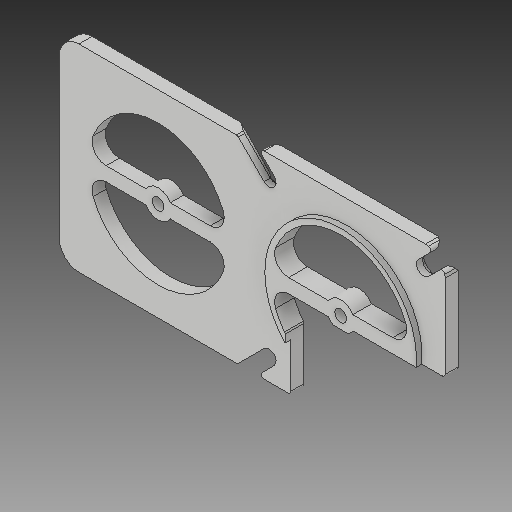
# Autodesk Inventor part: V4 in walldual
Saved by Autodesk Inventor 2020 (Build 240168000, 168)
## iProperties
Created: 2020-01-08
Part Number: V4 in walldual
Material: Generic
Document SubType Name: Modeling
Designer: user
Density: 1 g/cm^3
Appearance: Default
Author: user
Autodesk Inventor part; units mm, degrees
ref_plane "YZ Plane" through (0, 0, 0) normal (1, 0, 0) x (0, 1, 0)
ref_plane "XZ Plane" through (0, 0, 0) normal (0, 1, 0) x (-1, 0, 0)
ref_plane "XY Plane" through (0, 0, 0) normal (0, 0, 1) x (1, 0, 0)
sketch "Sketch1" plane through (0, 0, 0) normal (0, 0, 1) x (1, 0, 0)
  line L0 (-95.2, -35.2) -> (28.2, -35.2)
  line L1 (35.2, -28.2) -> (35.2, 28.2)
  line L2 (28.2, 35.2) -> (-95.2, 35.2)
  line L3 (-102.2, 28.2) -> (-102.2, -28.2)
  arc A0 (-95.2, 35.2) -> (-102.2, 28.2) centre (-95.2, 28.2) ccw
  arc A1 (35.2, 28.2) -> (28.2, 35.2) centre (28.2, 28.2) ccw
  arc A2 (-102.2, -28.2) -> (-95.2, -35.2) centre (-95.2, -28.2) ccw
  arc A3 (28.2, -35.2) -> (35.2, -28.2) centre (28.2, -28.2) ccw
  line L4 (24.8747, -2.5) -> (24.8747, 2.5) construction
  line L5 (-24.8747, 2.5) -> (-24.8747, -2.5) construction
  line L6 (24.8747, -2.5) -> (-24.8747, 2.5) construction
  line L7 (24.8747, 2.5) -> (-24.8747, -2.5) construction
  arc A4 (-23.1756, -9.375) -> (23.1756, -9.375) centre (0, 0) ccw
  arc A5 (23.1756, 9.375) -> (-23.1756, 9.375) centre (0, 0) ccw
  arc A6 (-18.5405, -2.5) -> (-23.1756, -9.375) centre (-18.5405, -7.5) ccw
  arc A7 (-23.1756, 9.375) -> (-18.5405, 2.5) centre (-18.5405, 7.5) ccw
  arc A8 (23.1756, -9.375) -> (18.5405, -2.5) centre (18.5405, -7.5) ccw
  arc A9 (18.5405, 2.5) -> (23.1756, 9.375) centre (18.5405, 7.5) ccw
  line L8 (-4.3301, 2.5) -> (-18.5405, 2.5)
  line L9 (-18.5405, -2.5) -> (-4.3301, -2.5)
  line L10 (4.3301, -2.5) -> (18.5405, -2.5)
  line L11 (18.5405, 2.5) -> (4.3301, 2.5)
  arc A10 (-4.3301, -2.5) -> (4.3301, -2.5) centre (0, 0) ccw
  arc A11 (4.3301, 2.5) -> (-4.3301, 2.5) centre (0, 0) ccw
  line L12 (-18.5405, 7.5) -> (18.5405, 7.5) construction
  line L13 (18.5405, -7.5) -> (-18.5405, -7.5) construction
  line L14 (0, 0) -> (0, -35.2) construction
  line L15 (0, 0) -> (0, 35.2) construction
  line L16 (0, 0) -> (35.2, 0) construction
  line L17 (-33.5, -35.2) -> (-33.5, 35.2) construction
  arc A12 (-90.1756, -9.375) -> (-43.8244, -9.375) centre (-67, 0) ccw
  arc A13 (-43.8244, 9.375) -> (-90.1756, 9.375) centre (-67, 0) ccw
  arc A14 (-43.8244, -9.375) -> (-48.4595, -2.5) centre (-48.4595, -7.5) ccw
  arc A15 (-48.4595, 2.5) -> (-43.8244, 9.375) centre (-48.4595, 7.5) ccw
  arc A16 (-85.5405, -2.5) -> (-90.1756, -9.375) centre (-85.5405, -7.5) ccw
  arc A17 (-90.1756, 9.375) -> (-85.5405, 2.5) centre (-85.5405, 7.5) ccw
  line L18 (-62.6699, 2.5) -> (-48.4595, 2.5)
  line L19 (-48.4595, -2.5) -> (-62.6699, -2.5)
  line L20 (-71.3301, -2.5) -> (-85.5405, -2.5)
  line L21 (-85.5405, 2.5) -> (-71.3301, 2.5)
  arc A18 (-71.3301, -2.5) -> (-62.6699, -2.5) centre (-67, 0) ccw
  arc A19 (-62.6699, 2.5) -> (-71.3301, 2.5) centre (-67, 0) ccw
  point P0 (0, 0)
  point P1 (0, 0)
  dimension "d63" = 67
  dimension "d1" = 7
  dimension "d3" = 5
  dimension "d4" = 25
  dimension "d5" = 5
  dimension "d7" = 5
  dimension "d59" = 70.4
  dimension "d60" = 137.4
  constraints: 44 end point, 44 point on circle, 20 centre point, 20 tangent, 18 symmetric about line, 7 equal radius, 7 midpoint, 7 parallel, 5 point on line, 4 horizontal, 3 coincident, 3 perpendicular, 2 equal length, 1 vertical, 9 other
  measures "d1" radius of A0
  measures "d3" distance of L5.end L5.start
  measures "d4" radius of A5
  measures "d5" radius of A6
  measures "d7" radius of A11
  measures "d59" distance between parallel lines of L0 L2
  measures "d60" distance between parallel lines of L3 L1
extrude "Extrusion1" add sketch "Sketch1" along normal blind 4.7
sketch "Sketch2" plane through (0, 0, 4.7) normal (0, 0, 1) x (1, 0, 0)
  circle A0 centre (0, 0) radius 27
  arc A1 (23.1756, 9.375) -> (-23.1756, 9.375) centre (0, 0) ccw projected
  arc A2 (18.5405, 2.5) -> (23.1756, 9.375) centre (18.5405, 7.5) ccw projected
  line L0 (18.5405, 2.5) -> (4.3301, 2.5) projected
  arc A3 (4.3301, 2.5) -> (-4.3301, 2.5) centre (0, 0) ccw projected
  line L1 (-4.3301, 2.5) -> (-18.5405, 2.5) projected
  arc A4 (-23.1756, 9.375) -> (-18.5405, 2.5) centre (-18.5405, 7.5) ccw projected
  line L2 (-18.5405, -2.5) -> (-4.3301, -2.5) projected
  arc A5 (-4.3301, -2.5) -> (4.3301, -2.5) centre (0, 0) ccw projected
  line L3 (4.3301, -2.5) -> (18.5405, -2.5) projected
  arc A6 (23.1756, -9.375) -> (18.5405, -2.5) centre (18.5405, -7.5) ccw projected
  arc A7 (-23.1756, -9.375) -> (23.1756, -9.375) centre (0, 0) ccw projected
  arc A8 (-18.5405, -2.5) -> (-23.1756, -9.375) centre (-18.5405, -7.5) ccw projected
  line L4 (28.2, 35.2) -> (-95.2, 35.2) projected
  arc A9 (-95.2, 35.2) -> (-102.2, 28.2) centre (-95.2, 28.2) ccw projected
  line L5 (-102.2, 28.2) -> (-102.2, -28.2) projected
  arc A10 (-102.2, -28.2) -> (-95.2, -35.2) centre (-95.2, -28.2) ccw projected
  line L6 (-95.2, -35.2) -> (28.2, -35.2) projected
  arc A11 (28.2, -35.2) -> (35.2, -28.2) centre (28.2, -28.2) ccw projected
  line L7 (35.2, -28.2) -> (35.2, 28.2) projected
  arc A12 (35.2, 28.2) -> (28.2, 35.2) centre (28.2, 28.2) ccw projected
  dimension "d10" = 54
  constraints: 1 centre point, 1 coincident
  measures "d10" diameter of A0
extrude "Extrusion2" add sketch "Sketch2" along normal blind 2 contours A0
sketch "Sketch3" plane through (0, 0, 0) normal (0, 0, -1) x (-1, 0, 0)
  line L0 (-27.5, -27.5) -> (27.5, -27.5) construction
  line L1 (27.5, -27.5) -> (27.5, 27.5) construction
  line L2 (27.5, 27.5) -> (-27.5, 27.5) construction
  line L3 (-27.5, 27.5) -> (-27.5, -27.5) construction
  line L4 (-27.5, -27.5) -> (27.5, 27.5) construction
  line L5 (27.5, -27.5) -> (-27.5, 27.5) construction
  line L6 (-27.5, 27.5) -> (-36.9678, 36.9678) construction
  line L7 (-25.7322, 29.2678) -> (-35.2, 38.7355)
  line L8 (-38.7355, 35.2) -> (-29.2678, 25.7322)
  arc A0 (-29.2678, 25.7322) -> (-25.7322, 29.2678) centre (-27.5, 27.5) ccw
  arc A1 (-35.2, 38.7355) -> (-38.7355, 35.2) centre (-36.9678, 36.9678) ccw
  line L9 (95.2, 35.2) -> (-28.2, 35.2) construction
  arc A2 (-38.7355, -35.2) -> (-35.2, -38.7355) centre (-36.9678, -36.9678) ccw
  line L10 (-29.2678, -25.7322) -> (-38.7355, -35.2)
  line L11 (-35.2, -38.7355) -> (-25.7322, -29.2678)
  arc A3 (-25.7322, -29.2678) -> (-29.2678, -25.7322) centre (-27.5, -27.5) ccw
  arc A4 (35.2, -38.7355) -> (38.7355, -35.2) centre (36.9678, -36.9678) ccw
  line L12 (25.7322, -29.2678) -> (35.2, -38.7355)
  line L13 (38.7355, -35.2) -> (29.2678, -25.7322)
  arc A5 (29.2678, -25.7322) -> (25.7322, -29.2678) centre (27.5, -27.5) ccw
  arc A6 (38.7355, 35.2) -> (35.2, 38.7355) centre (36.9678, 36.9678) ccw
  line L14 (29.2678, 25.7322) -> (38.7355, 35.2)
  line L15 (35.2, 38.7355) -> (25.7322, 29.2678)
  arc A7 (25.7322, 29.2678) -> (29.2678, 25.7322) centre (27.5, 27.5) ccw
  arc A8 (62.6699, -2.5) -> (71.3301, -2.5) centre (67, 0) ccw construction
  line L16 (67, 0) -> (0, 0) construction
  line L17 (134, 0) -> (67, 0) construction
  arc A9 (92.7322, 29.2678) -> (96.2678, 25.7322) centre (94.5, 27.5) ccw
  line L18 (96.2678, 25.7322) -> (105.7355, 35.2)
  arc A10 (105.7355, 35.2) -> (102.2, 38.7355) centre (103.9678, 36.9678) ccw
  line L19 (102.2, 38.7355) -> (92.7322, 29.2678)
  line L20 (28.2645, 35.2) -> (37.7322, 25.7322)
  arc A11 (37.7322, 25.7322) -> (41.2678, 29.2678) centre (39.5, 27.5) ccw
  line L21 (41.2678, 29.2678) -> (31.8, 38.7355)
  arc A12 (31.8, 38.7355) -> (28.2645, 35.2) centre (30.0322, 36.9678) ccw
  line L22 (31.8, -38.7355) -> (41.2678, -29.2678)
  arc A13 (41.2678, -29.2678) -> (37.7322, -25.7322) centre (39.5, -27.5) ccw
  line L23 (37.7322, -25.7322) -> (28.2645, -35.2)
  arc A14 (28.2645, -35.2) -> (31.8, -38.7355) centre (30.0322, -36.9678) ccw
  line L24 (105.7355, -35.2) -> (96.2678, -25.7322)
  arc A15 (96.2678, -25.7322) -> (92.7322, -29.2678) centre (94.5, -27.5) ccw
  line L25 (92.7322, -29.2678) -> (102.2, -38.7355)
  arc A16 (102.2, -38.7355) -> (105.7355, -35.2) centre (103.9678, -36.9678) ccw
  point P0 (-32.2339, 32.2339)
  point P1 (129.6699, -2.5)
  point P2 (138.3301, -2.5)
  dimension "d68" = 55
  dimension "d70" = 5
  dimension "d73" = 360
  dimension "d211" = 67
  dimension "d214" = 67
  dimension "d221" = 360
  constraints: 52 end point, 32 point on circle, 16 centre point, 4 tangent, 3 horizontal, 3 midpoint, 3 parallel, 2 perpendicular, 1 collinear, 1 point on line, 97 other
  measures "d68" distance of L1.end L2.end
  measures "d70" distance between parallel lines of L8 L7
  measures "d211" distance of L16.start L16.end
  measures "d214" distance of A8.start point (129.67, -2.5)
extrude "Extrusion3" cut sketch "Sketch3" against normal through all contours A0 L8 A1 L7 | L10 A3 L11 A2 | L12 L22 L13 A4 | L12 L23 L13 L22 | L12 A5 L13 L23 | L14 L21 L15 A6 | L14 L20 L15 L21 | L14 A7 L15 L20
chamfer "Chamfer1" distance 2.5 angle 45 12 edges at (28.3939, 31.9294, 0) (25.7322, 25.7322, 0) (31.9294, 28.3939, 0) (-28.6983, 32.2339, 0) (-25.7322, 25.7322, 0) (-34.0017, 30.4661, 0) (-25.7322, -25.7322, 0) (-34.0017, -30.4661, 0) (-28.6983, -32.2339, 0) (25.7322, -25.7322, 0) (28.3939, -31.9294, 0) (31.9294, -28.3939, 0)
fillet "Fillet1" radius 1 8 edges at (34.5911, -31.0555, 3.6) (31.0555, -34.5911, 3.6) (31.0555, 34.5911, 3.6) (34.5911, 31.0555, 3.6) (-31.6645, 35.2, 3.6) (-38.7355, 35.2, 3.6) (-31.6645, -35.2, 3.6) (-38.7355, -35.2, 3.6)
sketch "Sketch7" plane through (0, 0, 0) normal (0, 0, -1) x (-1, 0, 0)
  arc A0 (-4.3301, -2.5) -> (4.3301, -2.5) centre (0, 0) ccw construction
  arc A1 (62.6699, -2.5) -> (71.3301, -2.5) centre (67, 0) ccw projected
  point P0 (0, 0)
  constraints: 2 coincident
hole "Hole2" at (0, 0, 0) at (-67, 0, 0) direction (0, 0, 1) diameter 4.2 end through all
sketch "Sketch4" plane through (0, 0, 0) normal (0, 0, -1) x (-1, 0, 0)
  line L0 (19.8, -4.2) -> (19.8, -35.2)
  line L1 (19.8, -35.2) -> (-35.2, -35.2)
  line L2 (-35.2, -35.2) -> (-35.2, -4.2)
  line L3 (19.8, -4.2) -> (-35.2, -4.2)
  line L4 (102.2, -35.2) -> (-35.2, -35.2) construction
  line L5 (-35.2, -35.2) -> (-35.2, 35.2) construction
  line L6 (-35.2, 35.2) -> (102.2, 35.2) construction
  line L7 (102.2, 35.2) -> (102.2, -35.2) construction
  line L8 (28.1289, 35.2) -> (42.2711, 35.2) construction
  line L9 (-35.2, 28.1289) -> (-35.2, -28.1289) construction
  line L10 (-28.2, -35.2) -> (28.1289, -35.2) construction
  line L11 (102.2, -28.2) -> (102.2, 28.2) construction
  line L12 (-4.3301, -2.5) -> (-18.5405, -2.5) projected
  line L13 (-4.3301, -2.5) -> (-35.2, -2.5)
  line L14 (-35.2, -2.5) -> (-35.2, -4.2)
  line L15 (-35.2, -4.2) -> (-4.3301, -4.2)
  line L16 (-4.3301, -4.2) -> (-4.3301, -2.5)
  point P0 (-28.1289, 35.2)
  point P1 (-28.1289, -35.2)
  dimension "d39" = 31
  dimension "d41" = 55
  constraints: 24 end point, 4 collinear, 4 parallel, 4 perpendicular, 3 horizontal
  measures "d39" distance between parallel lines of L3 L1
  measures "d41" distance of L0.start L2.end
extrude "Extrusion4" cut sketch "Sketch4" against normal through all
fillet "Fillet2" radius 1 2 edges at (-19.8, -15.263, 3.35) (-19.8, -35.2, 2.35)
sketch "Sketch8" plane through (0, 0, 0) normal (0, 0, -1) x (-1, 0, 0)
  line L0 (0, 0) -> (35.5, 0) construction
  line L1 (35.5, 0) -> (71, 0) construction
  line L2 (32.5, 32.5) -> (32.5, -32.5) construction
  line L3 (32.5, -32.5) -> (-32.5, -32.5) construction
  line L4 (-32.5, -32.5) -> (-32.5, 32.5) construction
  line L5 (-32.5, 32.5) -> (32.5, 32.5) construction
  line L6 (99.5, 32.5) -> (99.5, -32.5) construction
  line L7 (99.5, -32.5) -> (34.5, -32.5) construction
  line L8 (34.5, -32.5) -> (34.5, 32.5) construction
  line L9 (34.5, 32.5) -> (99.5, 32.5) construction
  line L10 (96.3694, 32.5) -> (96.3694, 35.2) construction
  line L11 (99.5, 26.6962) -> (102.2, 26.6962) construction
  line L12 (92.7868, -32.5) -> (92.7868, -35.2) construction
  line L13 (102.2, -28.2) -> (102.2, 28.2) construction
  line L14 (42.2711, -35.2) -> (95.2, -35.2) construction
  line L15 (-35.2, -1.5) -> (-35.2, 28.2) construction
  line L16 (-35.2, 21.6184) -> (-32.5, 21.6184) construction
  line L17 (95.2, 35.2) -> (42.2711, 35.2) construction
  line L18 (29.4901, 25.1562) -> (37.9558, 25.1562)
  line L19 (37.9558, 25.1562) -> (37.9558, -3.6366)
  line L20 (37.9558, -3.6366) -> (29.4901, -3.6366)
  line L21 (29.4901, -3.6366) -> (29.4901, 25.1562)
  dimension "d131" = 65
  constraints: 20 end point, 8 equal length, 8 point on line, 4 horizontal, 2 perpendicular, 2 vertical, 1 collinear, 4 other
  measures "d131" distance of L3.end L4.end
extrude "Extrusion6" cut sketch "Sketch8" against normal blind 2
equation "\"Offset\" = 0.3"
equation "\"d56\" = 0.3"
body "Solid1"
